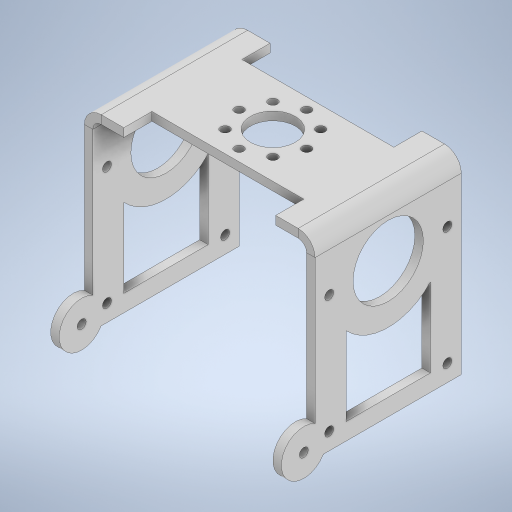
# Autodesk Inventor part: neck_bace
Saved by Autodesk Inventor 2024.1 (Build 281209000, 209)
## iProperties
Created: 2024-02-15
Part Number: neck_bace
Material: 一般
Document SubType Name: Sheet Metal
Designer: hibik
Density: 1 g/cm^3
Sheet Metal Rule: Default_mm
Appearance: 既定
Flat Pattern Width: 10.7786 cm
Flat Pattern Length: 3.2 cm
Flat Pattern Area: 34.4915 cm^2
Sheet Metal Width: 107.786 mm
Sheet Metal Length: 32.000 mm
Sheet Metal Area: 3449.147 mm^2
Author: hibik
Autodesk Inventor part; units mm, degrees
ref_plane "YZ Plane" through (0, 0, 0) normal (1, 0, 0) x (0, 1, 0)
ref_plane "XZ Plane" through (0, 0, 0) normal (0, 1, 0) x (-1, 0, 0)
ref_plane "XY Plane" through (0, 0, 0) normal (0, 0, 1) x (1, 0, 0)
sketch "スケッチ1" plane through (0, 0, 0) normal (0, 1, 0) x (-1, 0, 0)
  line L0 (20.5, -13) -> (-20.5, -13)
  line L1 (-20.5, -13) -> (-20.5, 13)
  line L2 (-20.5, 13) -> (20.5, 13)
  line L3 (20.5, 13) -> (20.5, -13)
  line L4 (20.5, -13) -> (-20.5, 13) construction
  line L5 (-20.5, -13) -> (20.5, 13) construction
  point P0 (0, 0)
  dimension "d0" = 41
  dimension "d1" = 26
  measures "d0" distance of L1.end L2.end
  measures "d1" distance of L0.end L1.end
extrude "プレート1" add sketch "スケッチ1" along normal blind 1.5
sketch "スケッチ2" plane through (19, 1.5, 13) normal (1, 0, 0) x (0, 1, 0)
  line L0 (0, -26) -> (0, 0)
  line L1 (0, 0) -> (-34, 0)
  line L2 (-34, 0) -> (-34, -26)
  line L3 (-34, -26) -> (0, -26)
  constraints: 6 end point, 1 horizontal, 1 perpendicular, 1 vertical
edge flange "フランジ1" height 34 angle 90 thickness 1.5 bend radius 1.5 thickness toward (1, 0, 0) relief straight relief width 1.5 relief depth 0.75 corner gap 1.5 corner form 0 edges at (20.5, 0, 0) (-20.5, 0, 0) wall of the first edge with corners at (19, 1.5, -13) (19, 1.5, 13) (19, -32.5, 13) (19, -32.5, -13)
bend "曲げ1"
corner "コーナー1"
sketch "スケッチ6" plane through (20.5, -32.5, 13) normal (1, 0, 0) x (0, 0, -1)
  line L0 (26, 0) -> (0, 0)
  line L1 (0, 0) -> (-4, 0)
  line L2 (-4, 0) -> (-4, 4)
  line L3 (-4, 4) -> (0, 4)
  line L4 (0, 4) -> (0, 0)
  circle A0 centre (-2, 2) radius 2
  circle A1 centre (-2, 2) radius 0.8
  circle A2 centre (-2, 2) radius 4
  line L5 (-5.4641, 0) -> (0, 0)
  point P0 (0, 31)
  point P1 (-2, 4)
  point P2 (-2, 0)
  point P3 (-4, 0)
  point P4 (1.4641, 0)
  dimension "d39" = 8
  dimension "d37" = 4
  dimension "d38" = 1.6
  measures "d37" diameter of A0
  measures "d38" diameter of A1
sheet face with bend "面2" sketch "スケッチ6" thickness 1.5 toward (-1, 0, 0) bend radius 1.5 relief straight relief width 1.5 relief depth 0.75
bend "曲げ2"
sketch "スケッチ7" plane through (20.5, -32.5, -13) normal (1, 0, 0) x (0, 0, -1)
  circle A0 centre (-13, 24) radius 6.25
  line L0 (0, 0) -> (-24.5359, 0) projected
  line L1 (-23.5, 24) -> (-2.5, 24) construction
  line L2 (-2.5, 24) -> (-2.5, 3) construction
  line L3 (-2.5, 3) -> (-23.5, 3) construction
  line L4 (-23.5, 3) -> (-23.5, 24) construction
  circle A1 centre (-23.5, 3) radius 0.8
  circle A2 centre (-2.5, 3) radius 0.8
  circle A3 centre (-23.5, 24) radius 0.8
  circle A4 centre (-2.5, 24) radius 0.8
  circle A5 centre (-13, 24) radius 10.25
  line L5 (-23.5, 24) -> (-2.5, 24)
  line L6 (-2.5, 24) -> (-2.5, 3) construction
  line L7 (-2.5, 3) -> (-23.5, 3)
  line L8 (-23.5, 3) -> (-23.5, 24) construction
  line L9 (-20.5, 17.0134) -> (-20.5, 3)
  line L10 (-5.5, 17.0134) -> (-5.5, 3)
  point P0 (-13, 32.5)
  point P1 (-26, 0)
  point P2 (-28, 0)
  point P3 (-31.4641, 0)
  dimension "d27" = 12.5
  dimension "d28" = 24
  dimension "d29" = 1.6
  dimension "d30" = 1.6
  dimension "d31" = 1.6
  dimension "d32" = 1.6
  dimension "d33" = 3
  dimension "d34" = 21
  dimension "d54" = 4
  dimension "d55" = 3
  dimension "d56" = 3
  constraints: 20 end point, 6 centre point, 5 coincident, 4 parallel, 2 horizontal, 2 perpendicular, 2 point on circle, 2 point on line, 2 vertical, 1 midpoint, 1 vertical alignment
  measures "d27" diameter of A0
  measures "d28" distance from line of A0.centre L0
  measures "d29" diameter of A1
  measures "d30" diameter of A2
  measures "d31" diameter of A3
  measures "d32" diameter of A4
  measures "d33" distance between parallel lines of L0 L3
  measures "d34" distance between parallel lines of L2 L4
  measures "d54" radial gap between concentric circles of A0 A5
  measures "d55" distance between parallel lines of L4 L9
  measures "d56" distance between parallel lines of L2 L10
extrude "切り取り4" cut sketch "スケッチ7" against normal blind 1.5 contours L5 A0 | A0 L5 | L5 A5 A4 | A4 A5 L5 | L5 A5 A3 | A3 A5 L5 | A4 A5 | A5 A3 | L10 L7 L9 A5 | A1 | A2
sketch "スケッチ8" plane through (0, 1.5, 0) normal (0, 1, 0) x (1, 0, 0)
  circle A0 centre (0, 0) radius 4
  circle A1 centre (0, 0) radius 6 construction
  circle A2 centre (0, 6) radius 0.8
  circle A3 centre (-4.2426, 4.2426) radius 0.8
  circle A4 centre (-6, 0) radius 0.8
  circle A5 centre (-4.2426, -4.2426) radius 0.8
  circle A6 centre (0, -6) radius 0.8
  circle A7 centre (4.2426, -4.2426) radius 0.8
  circle A8 centre (6, 0) radius 0.8
  circle A9 centre (4.2426, 4.2426) radius 0.8
  circle A10 centre (0, 0) radius 8
  line L0 (17.5, 13) -> (-17.5, 13) projected
  line L1 (-17.5, -13) -> (17.5, -13) projected
  line L2 (-13.5, 13) -> (13.5, 13)
  line L3 (13.5, 13) -> (13.5, -13)
  line L4 (13.5, -13) -> (-13.5, -13)
  line L5 (-13.5, -13) -> (-13.5, 13)
  line L6 (-17.5, 13) -> (-17.5, -13) projected
  line L7 (17.5, -13) -> (17.5, 13) projected
  line L8 (-13.5, 8) -> (13.5, 8)
  line L9 (13.5, 8) -> (13.5, -8)
  line L10 (13.5, -8) -> (-13.5, -8)
  line L11 (-13.5, -8) -> (-13.5, 8)
  line L12 (-13.5, 12) -> (13.5, 12)
  line L13 (13.5, 12) -> (13.5, 8)
  line L14 (13.5, 8) -> (-13.5, 8)
  line L15 (-13.5, 8) -> (-13.5, 12)
  line L16 (13.5, -8) -> (-13.5, -8)
  line L17 (-13.5, -8) -> (-13.5, -12)
  line L18 (-13.5, -12) -> (13.5, -12)
  line L19 (13.5, -12) -> (13.5, -8)
  point P0 (0, -8)
  point P1 (13.5, 8)
  point P2 (0, 8)
  point P3 (-13.5, -8)
  point P4 (-13.5, -13)
  dimension "d41" = 12
  dimension "d40" = 8
  dimension "d42" = 1.6
  dimension "d45" = 360
  dimension "d47" = 16
  dimension "d48" = 4
  dimension "d49" = 4
  dimension "d50" = 4
  dimension "d51" = 4
  constraints: 32 end point, 10 centre point, 8 parallel, 6 point on line, 4 coincident, 4 horizontal, 4 perpendicular, 2 tangent, 2 vertical alignment, 19 other
  measures "d40" diameter of A0
  measures "d42" diameter of A2
  measures "d47" diameter of A10
  measures "d48" distance between parallel lines of L5 L6
  measures "d49" distance between parallel lines of L7 L3
  measures "d50" distance between parallel lines of L14 L12
  measures "d51" distance between parallel lines of L18 L10
extrude "押し出し1" cut sketch "スケッチ8" against normal blind 1.5 contours A0 | A2 | A3 | A4 | A5 | A6 | A7 | A8 | A9 | L8 L5 L12 L3 | L10 L3 L18 L5 | L5 L0 L3 L12 | L3 L1 L5 L18
sketch "スケッチ9" plane through (-20.5, -32.5, -13) normal (-1, 0, 0) x (0, 0, 1)
  circle A0 centre (13, 24) radius 6.25 projected
  circle A1 centre (23.5, 24) radius 0.8 projected
  circle A2 centre (2.5, 3) radius 0.8 projected
  circle A3 centre (23.5, 3) radius 0.8 projected
  line L0 (5.5, 3) -> (20.5, 3) projected
  line L1 (20.5, 3) -> (20.5, 17.0134) projected
  arc A4 (5.5, 17.0134) -> (20.5, 17.0134) centre (13, 24) ccw projected
  line L2 (5.5, 17.0134) -> (5.5, 3) projected
  circle A5 centre (2.5, 24) radius 0.8 projected
  circle A6 centre (28, 2) radius 0.8 projected
  line L3 (0, 0) -> (24.5359, 0) projected
  line L4 (0, 31) -> (0, 0) projected
  line L5 (0, 31) -> (26, 31) projected
  line L6 (26, 5.4641) -> (26, 31) projected
  arc A7 (24.5359, 0) -> (26, 5.4641) centre (28, 2) ccw projected
  line L7 (26, 31) -> (0, 31) projected
  line L8 (0, 0) -> (0, 31) projected
  line L9 (26, 0) -> (0, 0) projected
  line L10 (26, 31) -> (26, 0) projected
  point P0 (13, 32.5)
sheet face with bend "面3" sketch "スケッチ9" thickness 1.5 toward (1, 0, 0) bend radius 1.5 relief straight relief width 1.5 relief depth 0.75 contours L9 L10 A7
bend "曲げ3"
extrude "切り取り5" cut sketch "スケッチ9" against normal blind 1.5 contours A0 | A1 | A2 | A3 | L2 A4 L1 L0 | A5
equation "\"d35\" = Thickness"
equation "\"d62\" = Thickness"
equation "\"d2\" = Thickness"
equation "\"d3\" = BendReliefWidth"
equation "\"d4\" = BendReliefDepth"
equation "\"d5\" = MinimumRemnant"
equation "\"d6\" = TransitionRadius"
equation "\"d9\" = BendRadius"
equation "\"d10\" = CornerReliefSize"
equation "\"d11\" = GapSize"
equation "\"d12\" = JacobiRadiusSize"
equation "\"d22\" = BendRadius"
equation "\"d23\" = BendReliefWidth"
equation "\"d25\" = MinimumRemnant"
equation "\"d24\" = BendReliefDepth"
equation "\"d26\" = TransitionRadius"
equation "\"d57\" = BendRadius"
equation "\"d58\" = BendReliefWidth"
equation "\"d60\" = MinimumRemnant"
equation "\"d59\" = BendReliefDepth"
equation "\"d61\" = TransitionRadius"
equation "\"BendRadius\" = Thickness"
equation "\"BendReliefWidth\" = Thickness"
equation "\"BendReliefDepth\" = 0.5 * Thickness"
equation "\"CornerReliefSize\" = 4 * Thickness"
equation "\"MinimumRemnant\" = 2 * Thickness"
equation "\"TransitionRadius\" = BendRadius"
equation "\"JacobiRadiusSize\" = BendRadius"
equation "\"GapSize\" = Thickness"
equation "\"Thickness\" = 1.5"
